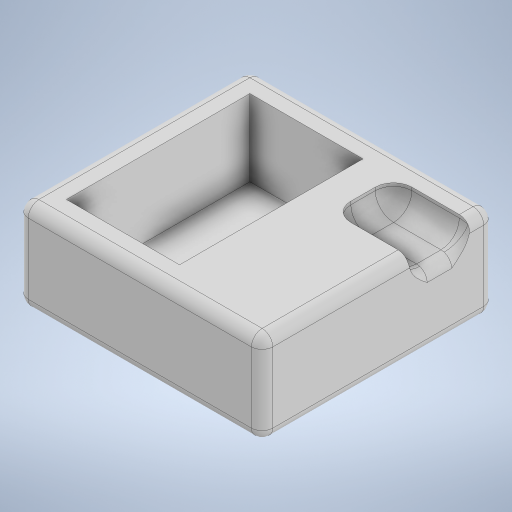
# Autodesk Inventor part: Wholeprototype
Saved by Autodesk Inventor 2023.6 (Build 276521000, 521)
## iProperties
Created: 2026-05-27
Part Number: Wholeprototype
Material: Generic
Document SubType Name: Modeling
Designer: Nanda
Density: 1 g/cm^3
Appearance: Default
Author: Nanda
Autodesk Inventor part; units mm, degrees
ref_plane "YZ Plane" through (0, 0, 0) normal (1, 0, 0) x (0, 1, 0)
ref_plane "XZ Plane" through (0, 0, 0) normal (0, 1, 0) x (-1, 0, 0)
ref_plane "XY Plane" through (0, 0, 0) normal (0, 0, 1) x (1, 0, 0)
sketch "Sketch1" plane through (0, 0, 0) normal (0, 1, 0) x (-1, 0, 0)
  line L0 (-50, -38) -> (30, -38)
  line L1 (30, -38) -> (30, 38)
  line L2 (30, 38) -> (-50, 38)
  line L3 (-50, 38) -> (-50, -38)
  line L4 (-50, -38) -> (30, 38) construction
  line L5 (30, -38) -> (-50, 38) construction
  point P0 (-10, 0)
  dimension "d2" = 80
  dimension "d3" = 76
  constraints: 12 end point, 2 midpoint, 2 parallel, 1 horizontal, 1 perpendicular
  measures "d2" distance of L2.end L1.end
  measures "d3" distance of L1.end L0.end
extrude "Extrusion1" add sketch "Sketch1" along normal blind 30
sketch "Sketch2" plane through (0, 30, 0) normal (0, 1, 0) x (1, 0, 0)
  line L0 (-30, 38) -> (-30, -38) construction
  line L1 (-30, 38) -> (-30, -38) projected
  line L2 (-30, -38) -> (50, -38) construction
  line L3 (-30, -38) -> (50, -38) projected
  line L4 (50, -38) -> (50, 38) construction
  line L5 (50, -38) -> (50, 38) projected
  line L6 (50, 38) -> (-30, 38) construction
  line L7 (50, 38) -> (-30, 38) projected
  line L8 (-22, -30) -> (15, -30)
  line L9 (-27.2231, 0) -> (28.9113, 0) construction
  line L10 (-22, 30) -> (15, 30)
  line L11 (-22, -30) -> (-22, 30)
  line L12 (15, 30) -> (15, -30)
  point P0 (0, 0)
  dimension "d6" = 76
  dimension "d7" = 37
  dimension "d8" = 8
  dimension "d9" = 8
  constraints: 10 end point, 2 horizontal, 2 symmetric about line, 1 parallel, 1 vertical
  measures "d6" distance of L0.start L0.end
  measures "d7" distance of L8.start L8.end
  measures "d8" distance between parallel lines of L8 L2
  measures "d9" distance from line of L0 L8.start
extrude "Extrusion2" cut sketch "Sketch2" against normal blind 25 contours L11 L10 L12 L8
sketch "Sketch3" plane through (50, 0, 38) normal (1, 0, 0) x (0, 0, -1)
  line L0 (0, 0) -> (0, 30) projected
  line L1 (0, 0) -> (0, 30) construction
  line L2 (8, 30) -> (8, 5) projected
  line L3 (8, 30) -> (8, 5) projected
  line L4 (0, 30) -> (76, 30) construction
  line L5 (0, 0) -> (76, 0) construction
  line L6 (76, 0) -> (76, 30) construction
  line L7 (68, 30) -> (8, 30) projected
  line L8 (68, 30) -> (68, 5) construction
  line L9 (68, 5) -> (8, 5) projected
  line L10 (76, 30) -> (0, 30) projected
  line L11 (76, 0) -> (0, 0) projected
  line L12 (76, 0) -> (76, 30) projected
  line L13 (8, 5) -> (68, 5) projected
  line L14 (8, 30) -> (68, 30) projected
  line L15 (68, 30) -> (68, 5) projected
  line L16 (68, 30) -> (68, 23)
  line L17 (68, 30) -> (75, 30) construction
  line L18 (68, 23) -> (48, 23)
  line L19 (68, 23) -> (88, 23) construction
  line L20 (48, 23) -> (48, 30)
  line L21 (48, 30) -> (68, 30)
  point P0 (38, 0)
  dimension "d12" = 7
  dimension "d13" = 90
  dimension "d15" = 20
  dimension "d16" = 180
  constraints: 12 end point, 3 horizontal, 2 equal length, 2 perpendicular, 2 point on line, 1 collinear
  measures "d12" distance of L16.start L16.end
  measures "d13" angle of L16 L17
  measures "d15" distance of L16.end L18.end
  measures "d16" angle of L18 L19
extrude "Extrusion3" cut sketch "Sketch3" against normal blind 25 contours L7 L15 L18 L20
fillet "Fillet1" radius 3.5 11 edges at (10, 30, -38) (-30, 30, 0) (10, 30, 38) (10, 0, -38) (-30, 15, -38) (-30, 0, 0) (-30, 15, 38) (10, 0, 38) (50, 15, 38) (50, 0, 0) (50, 30, 14)
fillet "Fillet2" radius 3.5 4 edges at (50, 28.9749, -36.9749) (50, 30, -32.25) (48.9749, 1.0251, -36.9749) (50, 15, -38)
fillet "Fillet3" radius 3.5 1 edges at (50, 23, -20)
fillet "Face Fillet1" radius 6 1 edges at (35.75, 23, -30)
fillet "Face Fillet2" radius 6 1 edges at (25, 23, -17)
fillet "Face Fillet3" radius 6 1 edges at (38.75, 23, -10)
body "Solid1"
